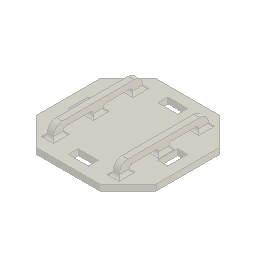
Bottom Plate (Autodesk Fusion 360 design; units mm, degrees)
Autodesk Fusion 360 part; units mm, degrees
sketch "Sketch1" plane through (0, 0, 0) normal (0, 0, 1) x (1, 0, 0)
  line L0 (0, 0) -> (60, 0)
  line L1 (60, 0) -> (60, 60)
  line L2 (60, 60) -> (0, 60)
  line L3 (0, 60) -> (0, 0)
  line L4 (0, 45.8579) -> (14.1421, 60)
  line L5 (0, 45.8579) -> (19.799, 45.8579) construction
  line L6 (14.1421, 0) -> (0, 14.1421)
  line L7 (14.1421, 0) -> (24.1421, 0) construction
  line L8 (60, 14.1421) -> (45.8579, 0)
  line L9 (60, 14.1421) -> (83.1045, 14.1421) construction
  line L10 (45.8579, 60) -> (60, 45.8579)
  line L11 (0, 30) -> (60, 30) construction
  line L12 (30, 60) -> (30, 0) construction
  line L13 (25, 55) -> (35, 55)
  line L14 (35, 55) -> (35, 50)
  line L15 (35, 50) -> (25, 50)
  line L16 (25, 50) -> (25, 55)
  line L17 (5, 25) -> (5, 35)
  line L18 (10, 35) -> (10, 25)
  line L19 (10, 25) -> (5, 25)
  line L20 (5, 35) -> (10, 35)
  line L21 (35, 5) -> (25, 5)
  line L22 (25, 10) -> (35, 10)
  line L23 (35, 10) -> (35, 5)
  line L24 (25, 5) -> (25, 10)
  line L25 (55, 35) -> (55, 25)
  line L26 (50, 25) -> (50, 35)
  line L27 (50, 35) -> (55, 35)
  line L28 (55, 25) -> (50, 25)
  point P0 (30, 30)
  dimension "d1" = 60
  dimension "d2" = 60
  dimension "d3" = 45
  dimension "d4" = 135
  dimension "d5" = 135
  dimension "d6" = 90
  dimension "d7" = 20
  dimension "d8" = 10
  dimension "d9" = 5
  dimension "d10" = 5
  dimension "d11" = 20
  dimension "d13" = 360
  constraint horizontal L0
  constraint vertical L1
  constraint horizontal L2
  constraint vertical L3
  constraint coincident L0.start L3.end
  constraint horizontal L5
  constraint coincident L3 L4.start
  constraint coincident L2 L4.end
  constraint horizontal L7
  constraint coincident L0 L6.start
  constraint coincident L3 L6.end
  constraint horizontal L9
  constraint coincident L1 L8.start
  constraint coincident L0 L8.end
  constraint coincident L2 L10.start
  constraint coincident L1 L10.end
  constraint equal L6 L10
  constraint equal L4 L8
  constraint equal L8 L10
  constraint midpoint L3 L11.start
  constraint midpoint L1 L11.end
  constraint midpoint L2 L12.start
  constraint midpoint L0 L12.end
  constraint midpoint L12 P0
  constraint horizontal L13
  constraint vertical L14
  constraint horizontal L15
  constraint vertical L16
  measures "d1" distance of L1 L3
  measures "d2" distance of L0.end L1.end
  measures "d3" angle of L4 L5
  measures "d4" angle of L6 L7
  measures "d5" angle of L8 L9
  measures "d6" angle of L8 L10
  measures "d7" distance of L10.start L10.end
  measures "d8" distance of L14.end L15.end
  measures "d9" distance of L12 L16
  measures "d10" distance of L13.end L14.end
  measures "d11" distance of L11 L15
extrude "Extrude1" add sketch "Sketch1" along normal blind 3 contours L0 L1 L2 L3 L4 L6 L8 L10
sketch "Sketch2" plane through (0, 0, 3) normal (0, 0, 1) x (-1, 0, 0)
  line L0 (-5, -25) -> (-5, -35)
  line L1 (-5, -35) -> (-10, -35)
  line L2 (-10, -35) -> (-10, -25)
  line L3 (-10, -25) -> (-5, -25)
  line L4 (-55, -35) -> (-55, -25)
  line L5 (-55, -25) -> (-50, -25)
  line L6 (-50, -25) -> (-50, -35)
  line L7 (-50, -35) -> (-55, -35)
  line L8 (-35, -5) -> (-25, -5)
  line L9 (-25, -5) -> (-25, -10)
  line L10 (-25, -10) -> (-35, -10)
  line L11 (-35, -10) -> (-35, -5)
  line L12 (-35, -50) -> (-25, -50)
  line L13 (-25, -50) -> (-25, -55)
  line L14 (-25, -55) -> (-35, -55)
  line L15 (-35, -55) -> (-35, -50)
  line L16 (0, -45.8579) -> (0, -14.1421)
  line L17 (0, -14.1421) -> (-14.1421, 0)
  line L18 (-14.1421, 0) -> (-45.8579, 0)
  line L19 (-45.8579, 0) -> (-60, -14.1421)
  line L20 (-60, -14.1421) -> (-60, -45.8579)
  line L21 (-60, -45.8579) -> (-45.8579, -60)
  line L22 (-45.8579, -60) -> (-14.1421, -60)
  line L23 (-14.1421, -60) -> (0, -45.8579)
ref_plane "WorkPlane1" through (30, 0, 0) normal (1, 0, 0) x (0, 1, 0)
sketch "Sketch3" plane through (30, 0, 0) normal (1, 0, 0) x (0, 1, 0)
  line L0 (52.5, 3) -> (7.5, 3)
  line L1 (7.5, 3) -> (7.5, 9)
  line L2 (7.5, 9) -> (52.5, 9)
  line L3 (52.5, 9) -> (52.5, 3)
  line L4 (47.5, 3) -> (32.5, 3)
  line L5 (32.5, 3) -> (32.5, 6)
  line L6 (32.5, 6) -> (47.5, 6)
  line L7 (47.5, 6) -> (47.5, 3)
  line L8 (27.5, 3) -> (12.5, 3)
  line L9 (12.5, 3) -> (12.5, 6)
  line L10 (12.5, 6) -> (27.5, 6)
  line L11 (27.5, 6) -> (27.5, 3)
  line L12 (60, 3) -> (0, 3)
  line L13 (0, 3) -> (0, 0)
  line L14 (0, 0) -> (60, 0)
  line L15 (60, 0) -> (60, 3)
  point P0 (30, 0)
  dimension "d17" = 45
  dimension "d18" = 6
  dimension "d21" = 3
  dimension "d22" = 5
  dimension "d23" = 5
  dimension "d24" = 5
  dimension "d25" = 22.5
  constraint horizontal L0
  constraint vertical L1
  constraint horizontal L2
  constraint vertical L3
  constraint horizontal L4
  constraint vertical L5
  constraint horizontal L6
  constraint vertical L7
  constraint coincident L0 L4.start
  constraint horizontal L8
  constraint vertical L9
  constraint horizontal L10
  constraint vertical L11
  constraint coincident L0 L8.start
  constraint equal L6 L10
  constraint horizontal L12
  constraint vertical L13
  constraint horizontal L14
  constraint vertical L15
  constraint coincident L13.end L14.start
  constraint midpoint L14 P0
  measures "d17" distance of L0.start L0.end
  measures "d18" distance of L0.start L2.end
  measures "d21" distance of L8.start L10.end
  measures "d22" distance of L3 L7
  measures "d23" distance of L1 L9
  measures "d24" distance of L5 L11
  measures "d25" distance of L3 P0
extrude "Extrude2" add sketch "Sketch3" along normal blind 3 from surface at 15 contours L0 L1 L2 L3 L5 L6 L7 L9 L10 L11 L12
extrude "Extrude3" add sketch "Sketch3" against normal blind 3 from surface at -15 contours L0 L1 L2 L3 L5 L6 L7 L9 L10 L11 L12
fillet "Fillet1" radius 1.5 24 edges at (13.5, 27.5, 3) (15, 30, 3) (13.5, 47.5, 3) (15, 50, 3) (13.5, 7.5, 3) (15, 10, 3) (46.5, 7.5, 3) (48, 10, 3) (46.5, 27.5, 3) (48, 30, 3) (46.5, 47.5, 3) (48, 50, 3) (46.5, 52.5, 3) (45, 50, 3) (46.5, 32.5, 3) (45, 30, 3) (46.5, 12.5, 3) (45, 10, 3) (13.5, 52.5, 3) (12, 50, 3) (13.5, 32.5, 3) (12, 30, 3) (13.5, 12.5, 3) (12, 10, 3)
fillet "Fillet1" radius 1.5 8 edges at (13.5, 12.5, 6) (13.5, 47.5, 6) (46.5, 27.5, 6) (46.5, 47.5, 6) (13.5, 27.5, 6) (13.5, 32.5, 6) (46.5, 32.5, 6) (46.5, 12.5, 6)
fillet "Fillet1" radius 4.5 4 edges at (13.5, 52.5, 9) (13.5, 7.5, 9) (46.5, 7.5, 9) (46.5, 52.5, 9)
equation "d1 = d2"
equation "d9 = d8 / 2"
equation "d23 = d22"
equation "d24 = d22"
equation "d25 = d17 / 2"
